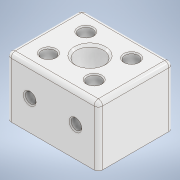
# Autodesk Inventor part: conector_ceramico
Saved by Autodesk Inventor 2021 (Build 250183000, 183)
## iProperties
Created: 2021-04-17
Part Number: conector_ceramico
Material: Porcelana, lino
Document SubType Name: Modeling
Designer: Leonardo Fabio Mercado Benítez
Density: 3.4 g/cm^3
Appearance: Topo pajizo
Mass: 15.2977 g
Surface Area: 23.8525 cm^2
Volume: 4.49931 cm^3
Author: Leonardo Fabio Mercado Benítez
Autodesk Inventor part; units mm, degrees
ref_plane "YZ Plane" through (0, 0, 0) normal (1, 0, 0) x (0, 1, 0)
ref_plane "XZ Plane" through (0, 0, 0) normal (0, 1, 0) x (-1, 0, 0)
ref_plane "XY Plane" through (0, 0, 0) normal (0, 0, 1) x (1, 0, 0)
sketch "Boceto1" plane through (0, 0, 0) normal (0, 1, 0) x (-1, 0, 0)
  line L0 (10.75, 8.8) -> (-10.75, 8.8)
  line L1 (-10.75, 8.8) -> (-10.75, -8.8)
  line L2 (-10.75, -8.8) -> (10.75, -8.8)
  line L3 (10.75, -8.8) -> (10.75, 8.8)
  line L4 (10.75, 8.8) -> (-10.75, -8.8) construction
  line L5 (-10.75, 8.8) -> (10.75, -8.8) construction
  point P0 (0, 0)
  dimension "d0" = 21.5
  dimension "d1" = 17.6
  constraints: 12 end point, 2 midpoint, 2 parallel, 1 horizontal, 1 perpendicular
  measures "d0" distance of L2.end L1.end
  measures "d1" distance of L1.end L0.end
extrude "Extrusión1" add sketch "Boceto1" along normal blind 14
sketch "Boceto2" plane through (0, 14, 0) normal (0, 1, 0) x (1, 0, 0)
  circle A0 centre (0, 0) radius 3.175
  point P0 (-10.75, -8.8)
  point P1 (10.75, -8.8)
  point P2 (10.75, 8.8)
  dimension "d9" = 6.35
  constraints: 1 centre point
  measures "d9" diameter of A0
extrude "Extrusión2" cut sketch "Boceto2" against normal up to surface (14 mm away)
chamfer "Chaflán1" distance 0.5 angle 45 1 edges at (-3.175, 14, 0)
sketch "Boceto3" plane through (-10.75, 0, 8.8) normal (0, 0, 1) x (1, 0, 0)
  line L0 (10.75, 0) -> (10.75, 14) construction
  line L1 (0, 14) -> (21.5, 14) construction
  line L2 (0, 14) -> (10.75, 0) construction
  line L3 (21.5, 0) -> (21.5, 14) construction
  line L4 (21.5, 13.961) -> (10.75, 0) construction
  line L5 (21.5, 0) -> (0, 0) construction
  line L6 (10.75, 14) -> (21.5, 0) construction
  line L7 (0, 0) -> (10.75, 14) construction
  circle A0 centre (5.375, 7) radius 1.25
  circle A1 centre (16.125, 7) radius 1.25
  dimension "d15" = 2.5
  dimension "d16" = 2.5
  constraints: 10 end point, 2 centre point, 2 midpoint, 1 parallel, 1 point on line, 1 vertical
  measures "d15" diameter of A0
  measures "d16" diameter of A1
sketch "Boceto4" plane through (0, 14, 0) normal (0, 1, 0) x (1, 0, 0)
  line L0 (-10.75, -8.8) -> (10.75, -8.8) construction
  line L1 (10.75, 8.8) -> (-10.75, 8.8) construction
  line L2 (-10.75, -8.8) -> (10.75, 8.8) construction
  line L3 (-10.75, 8.8) -> (-10.75, -8.8) construction
  line L4 (10.75, -8.8) -> (-10.75, 8.8) construction
  line L5 (0, -8.8) -> (-10.75, 0) construction
  line L6 (-10.75, 0) -> (0, 8.8) construction
  line L7 (0, -8.8) -> (10.75, 0) construction
  line L8 (10.75, -8.8) -> (10.75, 8.8) construction
  line L9 (10.75, 0) -> (0, 8.8) construction
  circle A0 centre (-5.375, -4.4) radius 1.5875
  circle A1 centre (-5.375, 4.4) radius 1.5875
  circle A2 centre (5.375, 4.4) radius 1.5875
  circle A3 centre (5.375, -4.4) radius 1.5875
  point P0 (0, 0)
  dimension "d17" = 3.175
  dimension "d18" = 3.175
  dimension "d19" = 3.175
  dimension "d20" = 3.175
  constraints: 12 end point, 8 midpoint, 4 centre point
  measures "d17" diameter of A0
  measures "d18" diameter of A1
  measures "d19" diameter of A2
  measures "d20" diameter of A3
sketch "Boceto5" plane through (10.75, 0, -8.8) normal (0, 0, -1) x (-1, 0, 0)
  line L0 (21.5, 14) -> (0, 14) construction
  line L1 (10.75, 14) -> (10.75, 0) construction
  line L2 (10.75, 0) -> (21.6018, 14) construction
  line L3 (0, 0) -> (21.5, 0) construction
  line L4 (10.75, 14) -> (21.5, 0) construction
  line L5 (0, 0) -> (10.75, 14) construction
  line L6 (0, 14) -> (10.75, 0) construction
  circle A0 centre (5.375, 7) radius 1.25
  circle A1 centre (16.125, 7) radius 1.25
  dimension "d21" = 2.5
  dimension "d22" = 2.5
  constraints: 10 end point, 3 midpoint, 2 centre point, 1 point on line, 1 vertical
  measures "d21" diameter of A0
  measures "d22" diameter of A1
extrude "Extrusión3" cut sketch "Boceto3" against normal blind 5.9875
extrude "Extrusión4" cut sketch "Boceto5" against normal blind 5.9875
extrude "Extrusión5" cut sketch "Boceto4" against normal blind 8.25
fillet "Empalme1" radius 1 8 edges at (10.75, 14, 0) (0, 14, 8.8) (0, 14, -8.8) (-10.75, 14, 0) (10.75, 7, 8.8) (10.75, 7, -8.8) (-10.75, 7, -8.8) (-10.75, 7, 8.8)
chamfer "Chaflán2" distance 0.25 angle 45 8 edges at (-6.9625, 14, -4.4) (3.7875, 14, -4.4) (3.7875, 14, 4.4) (-6.9625, 14, 4.4) (-6.625, 7, 8.8) (4.125, 7, 8.8) (-4.125, 7, -8.8) (6.625, 7, -8.8)
